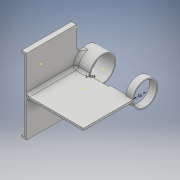
# Autodesk Inventor part: scopeHolder
Saved by Autodesk Inventor 2018 (Build 220112000, 112)
## iProperties
Created: 2019-03-14
Part Number: scopeHolder
Material: Generic
Document SubType Name: Modeling
Designer: Aditya Kendre
Density: 1 g/cm^3
Appearance: Default
Author: Aditya Kendre
Autodesk Inventor part; units mm, degrees
ref_plane "YZ Plane" through (0, 0, 0) normal (1, 0, 0) x (0, 1, 0)
ref_plane "XZ Plane" through (0, 0, 0) normal (0, 1, 0) x (-1, 0, 0)
ref_plane "XY Plane" through (0, 0, 0) normal (0, 0, 1) x (1, 0, 0)
sketch "Sketch1" plane through (0, 0, 0) normal (0, 1, 0) x (-1, 0, 0)
  line L0 (0, 0) -> (3, 0)
  line L1 (3, 0) -> (3, -100)
  line L2 (3, -100) -> (0, -100)
  line L3 (0, -100) -> (0, 0)
  dimension "d0" = 3
  dimension "d1" = 100
  constraints: 8 end point, 2 parallel, 1 horizontal, 1 perpendicular
  measures "d0" distance of L1.end L2.end
  measures "d1" distance of L0.end L1.end
extrude "Extrusion1" add sketch "Sketch1" along normal blind 70
sketch "Sketch2" plane through (-3, 0, 0) normal (0, 0, 1) x (1, 0, 0)
  line L0 (3, 0) -> (0, 0) projected
  line L1 (3, 0) -> (-4, 0)
  line L2 (-4, 0) -> (-4, 70)
  line L3 (-4, 70) -> (3, 70)
  line L4 (3, 70) -> (3, 0)
  dimension "d4" = 7
  constraints: 8 end point, 2 parallel, 1 horizontal, 1 perpendicular
  measures "d4" distance of L2.end L3.end
extrude "Extrusion2" add sketch "Sketch2" along normal blind 3
sketch "Sketch3" plane through (0, 0, -100) normal (0, 0, -1) x (-1, 0, 0)
  line L0 (0, 0) -> (0, 70) projected
  line L1 (7, 70) -> (7, 0) projected
  line L2 (0, 70) -> (7, 70)
  line L3 (7, 70) -> (7, 0)
  line L4 (7, 0) -> (0, 0)
  line L5 (0, 0) -> (0, 70)
  constraints: 8 end point, 2 parallel, 1 horizontal, 1 perpendicular
extrude "Extrusion3" add sketch "Sketch3" along normal blind 3
sketch "Sketch4" plane through (0, 70, 0) normal (0, 1, 0) x (1, 0, 0)
  line L0 (-3, 100) -> (-3, 0) construction
  line L1 (-3, 0) -> (-7, 0) construction
  line L2 (-3, 100) -> (-3, 0) construction
  line L3 (-3, 50) -> (0, 50) construction
  point P0 (0, 0)
  constraints: 4 end point, 1 horizontal, 1 midpoint, 1 vertical
sketch "Sketch5" plane through (0, 0, 3) normal (1, 0, 0) x (0, 0, -1)
  line L0 (106, 70) -> (53, 70) construction
  line L1 (103, 70) -> (3, 70) construction
  line L2 (3, 0) -> (103, 0) construction
  line L3 (53, 0) -> (53, 70) construction
  line L4 (53, 70) -> (53, 87) construction
  circle A0 centre (53, 87) radius 17
  circle A1 centre (53, 87) radius 18.5
  point P0 (0, 70)
  dimension "d9" = 17
  dimension "d10" = 34
  dimension "d11" = 37
  constraints: 6 end point, 2 centre point, 2 coincident, 2 midpoint, 2 perpendicular
  measures "d9" distance of L0.end L4.end
  measures "d10" diameter of A0
  measures "d11" diameter of A1
extrude "Extrusion4" add sketch "Sketch5" along normal blind 20 and the other way blind 3
fillet "Fillet1" radius 10 2 edges at (-1.5, 70, -57.2973) (-1.5, 70, -42.7027)
sketch "Sketch6" plane through (0, 0, 3) normal (1, 0, 0) x (0, 0, -1)
  arc A0 (35.0667, 82.4561) -> (70.9333, 82.4561) centre (53, 87) ccw construction
  line L0 (53, 68.5) -> (53, 0) construction
  line L1 (106, 0) -> (0, 0) construction
  line L2 (54.5, -0.0609) -> (51.5, -0.0609)
  line L3 (51.5, -0.0609) -> (51.5, 68.5609)
  line L4 (51.5, 68.5609) -> (54.5, 68.5609)
  line L5 (54.5, 68.5609) -> (54.5, -0.0609)
  line L6 (54.5, -0.0609) -> (51.5, 68.5609) construction
  line L7 (51.5, -0.0609) -> (54.5, 68.5609) construction
  point P0 (3, 0)
  point P1 (53, 34.25)
  dimension "d17" = 3
  constraints: 14 end point, 4 midpoint, 2 parallel, 2 point on circle, 1 horizontal, 1 perpendicular
  measures "d17" distance of L3.end L4.end
extrude "Extrusion5" add sketch "Sketch6" along normal blind 80
fillet "Fillet2" radius 4 6 edges at (0, 34.2805, -48.5) (10, 68.5609, -48.5) (0, 72.8732, -38.055) (0, 34.2805, -51.5) (0, 72.8732, -61.945) (10, 68.5609, -51.5)
sketch "Sketch7" plane through (20, 68.5609, -48.5) normal (0, 1, 0) x (1, 0, 0)
  line L0 (-23, -17) -> (0, -17) construction
  line L1 (-23, -17) -> (-73, -17) construction
  line L2 (-73, -17) -> (-73, 20) construction
  line L3 (-73, 20) -> (-23, 20) construction
  line L4 (-23, 20) -> (-23, -17) construction
  line L5 (-23, -17) -> (27, -17) construction
  line L6 (27, -17) -> (27, 20) construction
  line L7 (27, 20) -> (-23, 20) construction
  line L8 (-23, 20) -> (-23, -17) construction
  line L9 (-20, 3) -> (60, 3) projected
  line L10 (0, 0) -> (60, 0) projected
  line L11 (60, 3) -> (27, 3)
  line L12 (27, 3) -> (27, 0)
  line L13 (27, 0) -> (60, 0)
  line L14 (60, 0) -> (60, 3)
  point P0 (-20, -48.5)
  dimension "d21" = 50
  dimension "d22" = 50
  constraints: 24 end point, 6 parallel, 4 point on line, 3 horizontal, 3 perpendicular
  measures "d21" distance of L2.end L3.end
  measures "d22" distance of L7.end L6.end
extrude "Extrusion6" add sketch "Sketch7" along normal blind 2.439
sketch "Sketch8" plane through (80, 0, 3) normal (1, 0, 0) x (0, 0, -1)
  line L0 (54.5, 70.9999) -> (51.5, 70.9999) construction
  line L1 (53, 70.9999) -> (53, 86.9999) construction
  point P0 (3, 0)
  dimension "d25" = 16
  constraints: 2 end point, 1 midpoint, 1 vertical
  measures "d25" distance of L1.start L1.end
sketch "Sketch9" plane through (80, 0, 3) normal (1, 0, 0) x (0, 0, -1)
  point P0 (3, 0)
sketch "Sketch10" plane through (20, 0, 3) normal (1, 0, 0) x (0, 0, -1)
  circle A0 centre (53, 87) radius 17 construction
  line L0 (53, 70) -> (53, 68.5609) construction
  line L1 (51.5, 68.5609) -> (54.5, 68.5609) construction
  point P0 (3, 0)
  dimension "d26" = 1.4391
  constraints: 2 end point, 1 midpoint, 1 vertical alignment, 1 other
  measures "d26" distance of L0.start L0.end
sketch "Sketch11" plane through (80, 0, 3) normal (1, 0, 0) x (0, 0, -1)
  line L0 (54.5, 70.9999) -> (51.5, 70.9999) construction
  line L1 (53, 70.9999) -> (53, 86.9999) construction
  circle A0 centre (53, 86.9999) radius 16
  circle A1 centre (53, 86.9999) radius 17.5
  point P0 (3, 0)
  dimension "d27" = 16
  dimension "d28" = 32
  dimension "d29" = 35
  constraints: 2 centre point, 2 coincident, 2 end point, 1 midpoint, 1 vertical
  measures "d27" distance of L1.start L1.end
  measures "d28" diameter of A0
  measures "d29" diameter of A1
extrude "Extrusion7" add sketch "Sketch11" against normal blind 10
body "Solid1"
